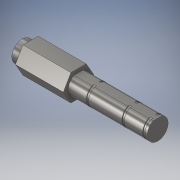
# Autodesk Inventor part: Gearbox Axle
Saved by Autodesk Inventor 2019.4 (Build 234330000, 330)
## iProperties
Created: 2020-01-18
Part Number: Gearbox Axle
Material: Steel, Mild
Document SubType Name: Modeling
Designer: admin
Density: 7.85 g/cm^3
Appearance: Semi-Polished
Mass: 42.1934 g
Surface Area: 24.3527 cm^2
Volume: 5.37496 cm^3
Author: admin
Autodesk Inventor part; units mm, degrees
ref_plane "YZ Plane" through (0, 0, 0) normal (1, 0, 0) x (0, 1, 0)
ref_plane "XZ Plane" through (0, 0, 0) normal (0, 1, 0) x (-1, 0, 0)
ref_plane "XY Plane" through (0, 0, 0) normal (0, 0, 1) x (1, 0, 0)
sketch "Sketch1" plane through (0, 0, 0) normal (0, 0, 1) x (1, 0, 0)
  line L0 (0, 0) -> (0, 5)
  line L1 (0, 5) -> (4, 5)
  line L2 (4, 5) -> (4, 8.89)
  line L3 (4, 8.89) -> (27.029, 8.89)
  line L4 (27.029, 8.89) -> (27.029, 5)
  line L5 (27.029, 5) -> (35.729, 5)
  line L6 (35.729, 5) -> (35.729, 4.65)
  line L7 (35.729, 4.65) -> (36.829, 4.65)
  line L8 (36.829, 4.65) -> (36.829, 5)
  line L9 (36.829, 5) -> (52.829, 5)
  line L10 (52.829, 5) -> (52.829, 4.65)
  line L11 (52.829, 4.65) -> (53.929, 4.65)
  line L12 (53.929, 4.65) -> (53.929, 5)
  line L13 (65.029, 5) -> (65.029, 0)
  line L14 (65.029, 0) -> (0, 0)
  line L15 (53.929, 5) -> (62.829, 5)
  line L16 (62.829, 5) -> (62.829, 4.65)
  line L17 (62.829, 4.65) -> (63.929, 4.65)
  line L18 (63.929, 4.65) -> (63.929, 5)
  line L19 (63.929, 5) -> (65.029, 5)
  dimension "d0" = 5
  dimension "d1" = 8.89
  dimension "d2" = 23.029
  dimension "d3" = 1.1
  dimension "d4" = 16
  dimension "d5" = 8.7
  dimension "d6" = 0.35
  dimension "d7" = 4
  dimension "d9" = 1.1
  dimension "d14" = 1.1
  dimension "d15" = 0.35
  dimension "d16" = 26
  dimension "d17" = 1.1
  constraints: 40 end point, 14 perpendicular, 8 point on line, 2 vertical, 1 horizontal
  measures "d0" distance between parallel lines of L14 L1
  measures "d1" distance between parallel lines of L14 L3
  measures "d2" distance of L2.end L3.end
  measures "d3" distance of L6.end L7.end
  measures "d4" distance of L8.end L9.end
  measures "d5" distance of L4.end L5.end
  measures "d6" distance of L5.end L6.end
  measures "d7" distance of L0.end L1.end
  measures "d9" distance of L10.end L11.end
  measures "d14" distance of L16.end L17.end
  measures "d15" distance of L17.end L18.end
  measures "d16" distance between parallel lines of L8 L16
  measures "d17" distance of L18.end L13.start
revolve "Revolution1" add sketch "Sketch1" angle 360 about axis through (65.029, 0, 0) along (-1, 0, 0)
sketch "Sketch2" plane through (27.029, 0, 0) normal (1, 0, 0) x (0, 0, -1)
  line L0 (-7.303, 0) -> (-3.6515, 6.3246)
  line L1 (-3.6515, 6.3246) -> (3.6515, 6.3246)
  line L2 (3.6515, 6.3246) -> (7.303, 0)
  line L3 (7.303, 0) -> (3.6515, -6.3246)
  line L4 (3.6515, -6.3246) -> (-3.6515, -6.3246)
  line L5 (-3.6515, -6.3246) -> (-7.303, 0)
  circle A0 centre (0, 0) radius 8.89 projected
  point P0 (0, 0)
  dimension "d11" = 12.6492
  constraints: 12 end point, 1 coincident, 1 horizontal, 13 other
  measures "d11" distance between parallel lines of L4 L1
extrude "Extrusion1" cut sketch "Sketch2" against normal through all
sketch "Sketch3" plane through (65.029, 0, 0) normal (1, 0, 0) x (0, 0, -1)
  circle A0 centre (0, 0) radius 5 projected
  line L0 (-2.1794, 4.5) -> (2.1794, 4.5)
  point P0 (0, 0)
  dimension "d18" = 4.5
  constraints: 2 end point, 2 point on circle, 1 horizontal
  measures "d18" distance from line of point (0, 0) L0
extrude "Extrusion2" cut sketch "Sketch3" against normal up to surface (38 mm away) contours L0 A0 picked at (0, 4.6667)
body "Solid1"
